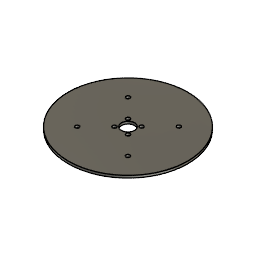
part - body adapter (Autodesk Fusion 360 design; units mm, degrees)
Autodesk Fusion 360 part; units mm, degrees
note: some values were not read from the file. Set by a fixed rule: which sketch regions a step uses.
sketch "Sketch1" plane through (0, 0, 0) normal (0, 0, 1) x (1, 0, 0)
  circle A0 centre (0, 0) radius 49.9
  circle A1 centre (-21.2132, 21.2132) radius 1.6
  line L0 (-21.2132, 21.2132) -> (0, 0)
  line L1 (0, 0) -> (-35.3413, 0)
  circle A2 centre (-21.2132, -21.2132) radius 1.6
  circle A3 centre (21.2132, -21.2132) radius 1.6
  circle A4 centre (21.2132, 21.2132) radius 1.6
  circle A5 centre (-5.6569, 5.6569) radius 1.6
  circle A6 centre (-5.6569, -5.6569) radius 1.6
  circle A7 centre (5.6569, -5.6569) radius 1.6
  circle A8 centre (5.6569, 5.6569) radius 1.6
  circle A9 centre (0, 0) radius 11.5
  circle A10 centre (0, 0) radius 5.5
  dimension "d1" = 99.8
  dimension "d2" = 3.2
  dimension "d3" = 45
  dimension "d4" = 30
  dimension "d6" = 360
  dimension "d7" = 3.2
  dimension "d8" = 8
  dimension "d9" = 23
  dimension "d14" = 11
  constraint coincident A0.centre L0.end
  constraint coincident A1.centre L0.start
  constraint horizontal L1
  constraint coincident L0 A5.centre
  measures "d1" diameter of A0
  measures "d2" diameter of A1
  measures "d3" angle of L0 L1
  measures "d4" distance of A1.centre A0.centre
  measures "d7" diameter of A5
  measures "d8" distance of A0.centre A5.centre
  measures "d9" diameter of A9
  measures "d14" diameter of A10
extrude "Extrude1" add sketch "Sketch1" along normal blind 2 contours A0 | L0 L1 A5 A9 A10 | L0 L1 A5 A9 A10 | L0 A5 | L0 A5 | L0 L1 A10 | L0 L1 A10 | A6 | A7 | A8
extrude "Extrude3" cut sketch "Sketch1" along normal blind 35 contours L0 A5 | L0 A5 | L0 L1 A10 | L0 L1 A10 | A6 | A7 | A8
